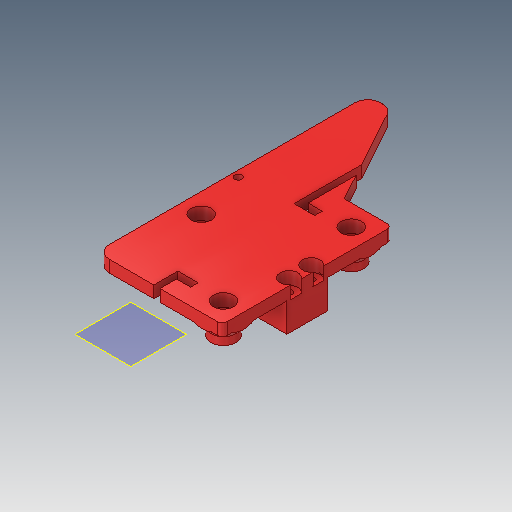
# Autodesk Inventor part: Neje_Base_Slide_y
Saved by Autodesk Inventor 2019.4 (Build 234330000, 330)
## iProperties
Created: 2021-04-08
Part Number: Neje_Base_Slide_y
Material: Generic
Document SubType Name: Modeling
Designer: diederichbenedict
Density: 1 g/cm^3
Appearance: Light Red
Mass: 28.126 g
Surface Area: 154.411 cm^2
Volume: 28.126 cm^3
Author: diederichbenedict
Autodesk Inventor part; units mm, degrees
sketch "Sketch1" plane through (0, 0, 0) normal (0, 1, 0) x (1, 0, 0)
  line L0 (-33.2203, 53.235) -> (-33.2203, 63.735)
  line L1 (-31.2203, 65.735) -> (-13.2203, 65.735)
  line L2 (-13.2203, 65.735) -> (-13.2203, 72.735)
  line L3 (-11.2203, 74.735) -> (-4.5203, 74.735)
  line L4 (-4.5203, 74.735) -> (-4.5203, 84.735)
  line L5 (-2.5203, 86.735) -> (14.3797, 86.735)
  line L6 (16.3797, 84.735) -> (16.3797, 67.935)
  arc A0 (16.3797, 84.735) -> (14.3797, 86.735) centre (14.3797, 84.735) ccw
  arc A1 (-2.5203, 86.735) -> (-4.5203, 84.735) centre (-2.5203, 84.735) ccw
  arc A2 (-11.2203, 74.735) -> (-13.2203, 72.735) centre (-11.2203, 72.735) ccw
  circle A3 centre (13.5797, 57.6229) radius 1.4
  circle A4 centre (8.5797, 78.435) radius 2.45
  circle A5 centre (-25.4203, 53.235) radius 2.45
  line L7 (16.3797, 53.235) -> (-22.9703, 53.235)
  line L8 (-27.8703, 53.235) -> (-33.2203, 53.235)
  arc A6 (-31.2203, 65.735) -> (-33.2203, 63.735) centre (-31.2203, 63.735) ccw
  line L9 (16.3797, 67.935) -> (16.3797, 53.235)
  point P0 (0, 0)
  point P1 (-33.2203, 65.735)
  dimension "d1" = 20
  dimension "d2" = 9
  dimension "d3" = 8.7
  dimension "d4" = 12
  dimension "d5" = 20.9
  dimension "d10" = 2.8
  dimension "d11" = 4.9
  dimension "d12" = 4.9
  dimension "d14" = 7.8
  dimension "d15" = 8.3
  dimension "d22" = 34
  dimension "d40" = 2
  constraints: 20 end point, 10 point on circle, 9 perpendicular, 8 tangent, 7 centre point, 2 equal radius, 2 horizontal, 2 point on line
  measures "d1" distance between parallel lines of L2 L0
  measures "d2" distance between parallel lines of L1 L3
  measures "d3" distance between parallel lines of L4 L2
  measures "d4" distance between parallel lines of L3 L5
  measures "d5" distance between parallel lines of L6 L4
  measures "d10" diameter of A3
  measures "d11" diameter of A4
  measures "d12" diameter of A5
  measures "d14" distance from line of A4.centre L6
  measures "d15" distance from line of A4.centre L5
  measures "d22" horizontal distance of A5.centre A4.centre
  measures "d40" radius of A6
extrude "Extrusion1" add sketch "Sketch1" along normal blind 4.7 contours L0 A6 L1 L2 A2 L3 L4 A1 L5 A0 L6 L9 L7 A5 L8
mirror "Mirror1" about plane through (-22.9703, 0, -53.235) normal (0, 0, 1) of "Extrusion1"
sketch "Sketch2" plane through (0, 0, 0) normal (0, -1, 0) x (-1, 0, 0)
  circle A0 centre (-8.5797, 28.035) radius 2.45 projected
  circle A1 centre (-8.5797, 78.435) radius 2.45 projected
  circle A2 centre (-8.5797, 28.035) radius 5
  circle A3 centre (-8.5797, 78.435) radius 5
  circle A4 centre (25.4203, 53.235) radius 2.45 projected
  circle A5 centre (25.4203, 53.235) radius 5
  point P0 (0, 0)
  dimension "d23" = 10
  dimension "d24" = 10
  dimension "d54" = 10
  constraints: 3 centre point, 3 coincident
  measures "d23" diameter of A2
  measures "d24" diameter of A3
  measures "d54" diameter of A5
extrude "Extrusion2" add sketch "Sketch2" along normal blind 7
chamfer "Chamfer1" distance 4 angle 45 3 edges at (13.5797, 0, -28.035) (13.5797, 0, -78.435) (-25.4203, 0, -58.235)
sketch "Sketch4" plane through (0, 4.7, 0) normal (0, 1, 0) x (1, 0, 0)
  circle A0 centre (8.5797, 28.035) radius 2.45 projected
  circle A1 centre (8.5797, 78.435) radius 2.45 projected
  circle A2 centre (-25.4203, 53.235) radius 2.45 projected
  circle A3 centre (8.5797, 28.035) radius 4
  circle A4 centre (-25.4203, 53.235) radius 4
  circle A5 centre (8.5797, 78.435) radius 4
  point P0 (0, 0)
  dimension "d41" = 8
  dimension "d42" = 8
  dimension "d43" = 8
  constraints: 3 centre point, 3 coincident
  measures "d41" diameter of A3
  measures "d42" diameter of A4
  measures "d43" diameter of A5
extrude "Extrusion4" cut sketch "Sketch4" against normal blind 5
sketch "Sketch5" plane through (0, 4.7, 0) normal (0, 1, 0) x (1, 0, 0)
  circle A0 centre (8.5797, 78.435) radius 4 projected
  circle A1 centre (8.5797, 28.035) radius 4 projected
  circle A2 centre (-25.4203, 53.235) radius 4 projected
  arc A3 (16.3797, 84.735) -> (14.3797, 86.735) centre (14.3797, 84.735) ccw projected
  line L0 (14.3797, 86.735) -> (-2.5203, 86.735) projected
  arc A4 (-2.5203, 86.735) -> (-4.5203, 84.735) centre (-2.5203, 84.735) ccw projected
  line L1 (-4.5203, 84.735) -> (-4.5203, 74.735) projected
  line L2 (-4.5203, 74.735) -> (-11.2203, 74.735) projected
  arc A5 (-11.2203, 74.735) -> (-13.2203, 72.735) centre (-11.2203, 72.735) ccw projected
  line L3 (-13.2203, 72.735) -> (-13.2203, 65.735) projected
  line L4 (-13.2203, 65.735) -> (-31.2203, 65.735) projected
  arc A6 (-31.2203, 65.735) -> (-33.2203, 63.735) centre (-31.2203, 63.735) ccw projected
  line L5 (-33.2203, 63.735) -> (-33.2203, 42.735) projected
  arc A7 (-33.2203, 42.735) -> (-31.2203, 40.735) centre (-31.2203, 42.735) ccw projected
  line L6 (-13.2203, 40.735) -> (-31.2203, 40.735) projected
  line L7 (-13.2203, 33.735) -> (-13.2203, 40.735) projected
  arc A8 (-13.2203, 33.735) -> (-11.2203, 31.735) centre (-11.2203, 33.735) ccw projected
  line L8 (-4.5203, 31.735) -> (-11.2203, 31.735) projected
  line L9 (-4.5203, 21.735) -> (-4.5203, 31.735) projected
  arc A9 (-4.5203, 21.735) -> (-2.5203, 19.735) centre (-2.5203, 21.735) ccw projected
  line L10 (14.3797, 19.735) -> (-2.5203, 19.735) projected
  arc A10 (14.3797, 19.735) -> (16.3797, 21.735) centre (14.3797, 21.735) ccw projected
  circle A11 centre (13.5797, 48.8472) radius 1.4 projected
  circle A12 centre (13.5797, 57.6229) radius 1.4 projected
  circle A13 centre (-2.5203, 119.7519) radius 2.95
  circle A14 centre (6.8956, 28.235) radius 2.95
  line L11 (-13.2203, 72.735) -> (-13.2203, 65.735) projected
  line L12 (-24.344, 126.6691) -> (-33.2203, 126.6691)
  line L13 (-33.2203, 126.6691) -> (-33.2203, 19.735)
  line L14 (-33.2203, 19.735) -> (-2.5203, 19.735)
  line L15 (16.3797, 84.735) -> (16.3797, 21.735) projected
  line L16 (-2.5203, 86.735) -> (-24.344, 126.6691)
  point P0 (0, 0)
  dimension "d46" = 5.9
  dimension "d47" = 5.9
  dimension "d88" = 25
  dimension "d90" = 92
  constraints: 8 end point, 2 centre point, 1 perpendicular, 1 point on circle, 1 point on line
  measures "d46" diameter of A13
  measures "d47" diameter of A14
  measures "d88" vertical distance of A14.centre A2.centre
  measures "d90" distance of A14.centre A13.centre
extrude "Extrusion5" add sketch "Sketch5" against normal up to surface (4.7 mm away) contours A4 L1 L2 A5 L3 L4 A6 L13 L12 L16 | L14 L13 A7 L6 L7 A8 L8 L9 A9
fillet "Fillet1" radius 5 3 edges at (-33.2203, 2.35, -19.735) (-33.2203, 2.35, -126.6691) (-24.344, 2.35, -126.6691)
sketch "Sketch6" plane through (0, 0, 0) normal (0, -1, 0) x (-1, 0, 0)
  circle A0 centre (27.2203, 28.235) radius 2.95 projected
  line L0 (-14.3797, 19.735) -> (28.2203, 19.735) projected
  line L1 (18.39, 19.735) -> (18.39, 34.735)
  line L2 (18.39, 34.735) -> (33.2203, 34.735)
  arc A1 (28.2203, 19.735) -> (33.2203, 24.735) centre (28.2203, 24.735) ccw projected
  line L3 (18.39, 19.735) -> (28.2203, 19.735)
  line L4 (33.2203, 34.735) -> (33.2203, 24.735)
  arc A2 (28.2203, 19.735) -> (33.2203, 24.735) centre (28.2203, 24.735) ccw
  circle A3 centre (26.4203, 53.235) radius 2.5
  line L5 (-16.3797, 84.735) -> (-16.3797, 21.735) projected
  line L6 (-2.3797, 61.235) -> (-16.3797, 61.235)
  line L7 (-16.3797, 61.235) -> (-16.3797, 45.235)
  line L8 (-16.3797, 45.235) -> (-2.3797, 45.235)
  line L9 (-2.3797, 45.235) -> (-2.3797, 61.235)
  line L10 (-2.3797, 61.235) -> (-16.3797, 45.235) construction
  line L11 (-16.3797, 61.235) -> (-2.3797, 45.235) construction
  circle A4 centre (-13.5797, 57.6229) radius 1.6 construction
  circle A5 centre (-13.5797, 48.8472) radius 1.4 projected
  line L12 (33.2203, 111.3869) -> (15.9923, 111.3869)
  line L13 (22.9219, 124.0669) -> (2.5203, 86.735) projected
  circle A6 centre (27.2203, 120.235) radius 2.95 projected
  line L14 (33.2203, 24.735) -> (33.2203, 121.6691) projected
  line L15 (33.2203, 111.3869) -> (33.2203, 121.6691)
  line L16 (15.9923, 111.3869) -> (22.9219, 124.0669)
  arc A7 (33.2203, 121.6691) -> (22.9219, 124.0669) centre (27.6842, 121.2067) ccw
  circle A8 centre (-13.5797, 57.6229) radius 1.4
  point P0 (0, 0)
  point P1 (33.2203, 48.745)
  point P2 (-9.3797, 53.235)
  dimension "d58" = 15
  dimension "d67" = 16
  dimension "d68" = 14
  dimension "d69" = 0
  dimension "d95" = 2.8
  constraints: 26 end point, 5 centre point, 4 point on circle, 3 horizontal, 3 point on line, 2 midpoint, 2 parallel, 2 perpendicular, 2 tangent, 1 coincident, 1 collinear, 1 concentric, 1 vertical, 4 other
  measures "d58" distance between parallel lines of L0 L2
  measures "d67" distance between parallel lines of L6 L8
  measures "d68" distance between parallel lines of L9 L7
  measures "d69" vertical distance of point (-9.38, 53.235) A3.centre
  measures "d95" diameter of A8
ref_plane "Work Plane2" through (-58.9603, 44.9175, -12.5) normal (0, 0, 1) x (0.8824126, -0.4704764, 0)
ref_plane "Work Plane6" through (-6.0157, -11.4, -93.0305) normal (0, -1, 0) x (0.9973542, 0, 0.0726957)
extrude "Extrusion6" add sketch "Sketch6" along normal up to surface (11.4 mm away) contours L6 L9 L8 L5
ref_plane "Work Plane3" through (-28.5805, 82.6129, 2.7) normal (0, 0, 1) x (0.7510442, -0.660252, 0)
ref_plane "Work Plane4" through (0, 3, 0) normal (0, -1, 0) x (-1, 0, 0)
sketch "Sketch11" plane through (0, 4.7, 0) normal (0, 1, 0) x (1, 0, 0)
  line L0 (-2.6203, -84.213) -> (-2.6203, 115.787) construction
  line L1 (-10.6203, -84.213) -> (-10.6203, 115.787) construction
  line L2 (5.0998, 19.735) -> (-28.2203, 19.735) projected
  line L3 (-10.6203, 19.735) -> (-8.1895, 19.735)
  line L4 (-8.1895, 19.735) -> (-8.1895, 26.2358)
  line L5 (-8.1895, 26.2358) -> (-10.6203, 26.2358)
  line L6 (-10.6203, 26.2358) -> (-10.6203, 19.735)
  line L7 (-10.6203, 26.2358) -> (-2.6203, 26.2358)
  line L8 (-2.6203, 26.2358) -> (-2.6203, 29.2358)
  line L9 (-2.6203, 29.2358) -> (-10.6203, 29.2358)
  line L10 (-10.6203, 29.2358) -> (-10.6203, 26.2358)
  line L11 (-10.7533, 102.8634) -> (-8.1895, 102.8634)
  line L12 (-8.1895, 102.8634) -> (-8.1895, 78.1694)
  line L13 (-8.1895, 78.1694) -> (-10.7533, 78.1694)
  line L14 (-10.7533, 78.1694) -> (-10.7533, 102.8634)
  line L15 (-10.7533, 78.1694) -> (-2.6203, 78.1694)
  line L16 (-2.6203, 78.1694) -> (-2.6203, 75.1694)
  line L17 (-2.6203, 75.1694) -> (-10.7533, 75.1694)
  line L18 (-10.7533, 75.1694) -> (-10.7533, 78.1694)
  point P0 (0, 0)
  point P1 (-18.39, 19.735)
  dimension "d77" = 0
  dimension "d78" = 3
  dimension "d79" = 3
  constraints: 36 end point, 8 parallel, 4 horizontal, 4 perpendicular, 4 point on line, 2 vertical, 4 other
  measures "d77" distance between parallel lines of L4 L12
  measures "d78" distance between parallel lines of L17 L15
  measures "d79" distance between parallel lines of L7 L9
extrude "Extrusion11" cut sketch "Sketch11" against normal blind 7
sketch "Sketch13" plane through (0, 4.7, 0) normal (0, 1, 0) x (1, 0, 0)
  circle A0 centre (13.5797, 48.8472) radius 1.4 projected
  circle A1 centre (13.5797, 57.6229) radius 1.4 projected
  circle A2 centre (13.5797, 48.8472) radius 3.5
  circle A3 centre (13.5797, 57.6229) radius 3.5
  point P0 (0, 0)
  dimension "d80" = 7
  dimension "d81" = 7
  constraints: 2 centre point, 2 coincident
  measures "d80" diameter of A2
  measures "d81" diameter of A3
extrude "Extrusion12" cut sketch "Sketch13" against normal blind 5
sketch "Sketch14" plane through (0, 4.7, 0) normal (0, 1, 0) x (1, 0, 0)
  arc A0 (16.3797, 59.7229) -> (16.3797, 55.5229) centre (13.5797, 57.6229) ccw projected
  arc A1 (16.3797, 50.9472) -> (16.3797, 46.7472) centre (13.5797, 48.8472) ccw projected
  circle A2 centre (-25.4203, 53.235) radius 4 projected
  circle A3 centre (8.5797, 28.035) radius 4 projected
  circle A4 centre (8.5797, 78.435) radius 4 projected
  line L0 (-10.6203, 19.735) -> (-10.6203, 29.2358) projected
  line L1 (-10.6203, 29.2358) -> (-2.6203, 29.2358) projected
  line L2 (-2.6203, 29.2358) -> (-2.6203, 26.2358) projected
  line L3 (-2.6203, 26.2358) -> (-8.1895, 26.2358) projected
  line L4 (-8.1895, 26.2358) -> (-8.1895, 19.735) projected
  line L5 (14.3797, 19.735) -> (-8.1895, 19.735) projected
  arc A5 (14.3797, 19.735) -> (16.3797, 21.735) centre (14.3797, 21.735) ccw projected
  line L6 (16.3797, 84.735) -> (16.3797, 59.7229) projected
  arc A6 (16.3797, 84.735) -> (14.3797, 86.735) centre (14.3797, 84.735) ccw projected
  line L7 (14.3797, 86.735) -> (-2.5203, 86.735) projected
  line L8 (-8.1895, 97.1089) -> (-2.5203, 86.735) projected
  line L9 (-8.1895, 97.1089) -> (-8.1895, 78.1694) projected
  line L10 (-8.1895, 78.1694) -> (-2.6203, 78.1694) projected
  line L11 (-2.6203, 78.1694) -> (-2.6203, 75.1694) projected
  line L12 (-2.6203, 75.1694) -> (-10.7533, 75.1694) projected
  line L13 (-10.7533, 75.1694) -> (-10.7533, 101.8003) projected
  line L14 (-22.9219, 124.0669) -> (-10.7533, 101.8003) projected
  arc A7 (-22.9219, 124.0669) -> (-27.3094, 126.6691) centre (-27.3094, 121.6691) ccw projected
  line L15 (-28.2203, 126.6691) -> (-27.3094, 126.6691) projected
  arc A8 (-28.2203, 126.6691) -> (-33.2203, 121.6691) centre (-28.2203, 121.6691) ccw projected
  line L16 (-33.2203, 24.735) -> (-33.2203, 121.6691) projected
  arc A9 (-33.2203, 24.735) -> (-28.2203, 19.735) centre (-28.2203, 24.735) ccw projected
  line L17 (-10.6203, 19.735) -> (-28.2203, 19.735) projected
  circle A10 centre (-30.8182, 73.2021) radius 1.45
  line L18 (16.3797, 46.7472) -> (16.3797, 21.735) projected
  line L19 (16.3797, 55.5229) -> (16.3797, 50.9472) projected
  point P0 (0, 0)
  dimension "d84" = 2.9
  constraints: 1 centre point
  measures "d84" diameter of A10
extrude "Extrusion13" cut sketch "Sketch14" against normal through all contours A10
ref_plane "Work Plane5" through (-40.8241, -11.4, -69.6389) normal (0, 1, 0) x (0.2292661, 0, 0.9733638)
sketch "Sketch15" plane through (0, 0, 0) normal (0, -1, 0) x (1, 0, 0)
  circle A0 centre (-30.8182, -73.2021) radius 1.45 projected
  line L0 (-10.6203, -29.2358) -> (-10.6203, -19.735) projected
  line L1 (-10.6203, -19.735) -> (-28.2203, -19.735) projected
  arc A1 (-28.2203, -19.735) -> (-33.2203, -24.735) centre (-28.2203, -24.735) ccw projected
  line L2 (-33.2203, -48.745) -> (-33.2203, -24.735) projected
  arc A2 (-33.2203, -57.725) -> (-33.2203, -48.745) centre (-25.4203, -53.235) ccw projected
  line L3 (-33.2203, -121.6691) -> (-33.2203, -57.725) projected
  arc A3 (-33.2203, -121.6691) -> (-28.2203, -126.6691) centre (-28.2203, -121.6691) ccw projected
  line L4 (-27.3094, -126.6691) -> (-28.2203, -126.6691) projected
  arc A4 (-27.3094, -126.6691) -> (-22.9219, -124.0669) centre (-27.3094, -121.6691) ccw projected
  line L5 (-10.7533, -101.8003) -> (-22.9219, -124.0669) projected
  line L6 (-10.7533, -101.8003) -> (-10.7533, -75.1694) projected
  line L7 (-10.7533, -75.1694) -> (-2.6203, -75.1694) projected
  line L8 (-2.6203, -75.1694) -> (-2.6203, -78.1694) projected
  line L9 (-2.6203, -78.1694) -> (-8.1895, -78.1694) projected
  line L10 (-8.1895, -78.1694) -> (-8.1895, -97.1089) projected
  line L11 (-2.5203, -86.735) -> (-8.1895, -97.1089) projected
  line L12 (5.0998, -86.735) -> (-2.5203, -86.735) projected
  arc A5 (16.3797, -73.945) -> (5.0998, -86.735) centre (8.5797, -78.435) ccw projected
  line L13 (16.3797, -61.235) -> (16.3797, -73.945) projected
  line L14 (16.3797, -32.525) -> (16.3797, -45.235) projected
  arc A6 (5.0998, -19.735) -> (16.3797, -32.525) centre (8.5797, -28.035) ccw projected
  line L15 (5.0998, -19.735) -> (-8.1895, -19.735) projected
  line L16 (-8.1895, -19.735) -> (-8.1895, -26.2358) projected
  line L17 (-8.1895, -26.2358) -> (-2.6203, -26.2358) projected
  line L18 (-2.6203, -26.2358) -> (-2.6203, -29.2358) projected
  line L19 (-2.6203, -29.2358) -> (-10.6203, -29.2358) projected
  line L20 (-10.7533, -101.8003) -> (-22.9219, -124.0669) projected
  line L21 (-20.6244, -119.8629) -> (-20.6244, -106.3025)
  line L22 (-20.6244, -106.3025) -> (-33.2203, -106.3025)
  line L23 (-33.2203, -121.6691) -> (-33.2203, -57.725) projected
  line L24 (-10.6203, -19.735) -> (-28.2203, -19.735) projected
  line L25 (-22.9219, -19.735) -> (-22.9219, -37.341)
  line L26 (-22.9219, -37.341) -> (-33.2203, -37.341)
  line L27 (-33.2203, -48.745) -> (-33.2203, -24.735) projected
  arc A7 (12.0597, -86.735) -> (16.3797, -82.925) centre (8.5797, -78.435) ccw projected
  line L28 (14.3797, -86.735) -> (12.0597, -86.735) projected
  arc A8 (14.3797, -86.735) -> (16.3797, -84.735) centre (14.3797, -84.735) ccw projected
  line L29 (16.3797, -82.925) -> (16.3797, -84.735) projected
  arc A9 (16.3797, -23.545) -> (12.0597, -19.735) centre (8.5797, -28.035) ccw projected
  arc A10 (16.3797, -21.735) -> (14.3797, -19.735) centre (14.3797, -21.735) ccw projected
  line L30 (14.3797, -19.735) -> (12.0597, -19.735) projected
  line L31 (16.3797, -21.735) -> (16.3797, -23.545) projected
  line L32 (16.3797, -61.235) -> (2.3797, -61.235) projected
  line L33 (2.3797, -61.235) -> (2.3797, -45.235) projected
  line L34 (2.3797, -45.235) -> (16.3797, -45.235) projected
  point P0 (0, 0)
  dimension "d91" = 90
  dimension "d92" = 90
  constraints: 8 end point, 4 point on line, 1 perpendicular, 1 vertical
  measures "d91" angle of L22 L21
  measures "d92" angle of L25 L26
extrude "Extrusion14" [suppressed]
body "Solid1"
